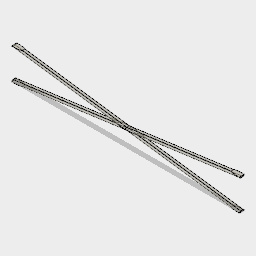
Cross braces (Autodesk Fusion 360 design; units mm, degrees)
Autodesk Fusion 360 part; units mm, degrees
sketch "Sketch1" plane through (0, 0, 0) normal (0, 0, 1) x (1, 0, 0)
  line L0 (457.0672, 59.1881) -> (558.2158, 72.9956)
  line L1 (456.2083, 65.4798) -> (534.7411, 76.2)
  line L2 (457.0672, 59.1881) -> (23.4747, 0)
  line L3 (456.2083, 65.4798) -> (0, 3.2044)
  line L4 (229.1567, 48.1231) -> (23.4747, 76.2)
  line L5 (228.2978, 41.8315) -> (0, 72.9956)
  line L6 (229.1567, 48.1231) -> (558.2158, 3.2044)
  line L7 (228.2978, 41.8315) -> (534.7411, 0)
  line L8 (23.4747, 76.2) -> (0, 76.2)
  line L9 (0, 76.2) -> (0, 72.9956)
  line L10 (0, 3.2044) -> (0, 0)
  line L11 (0, 0) -> (23.4747, 0)
  line L12 (534.7411, 76.2) -> (558.2158, 76.2)
  line L13 (558.2158, 76.2) -> (558.2158, 72.9956)
  line L14 (558.2158, 3.2044) -> (558.2158, 0)
  line L15 (558.2158, 0) -> (534.7411, 0)
  dimension "d1" = 558.2158
  dimension "d2" = 76.2
  measures "d1" distance of L10.end L14.end
  measures "d2" distance of L10.end L8.end
extrude "Extrude1" add sketch "Sketch1" along normal blind 12.7
fillet "Fillet1" radius 3.175 8 edges at (406.9245, 58.7522, 12.7) (430.3992, 20.6522, 12.7) (151.2913, 58.7522, 12.7) (430.3992, 55.5478, 12.7) (406.9245, 17.4478, 12.7) (151.2913, 17.4478, 12.7) (127.8166, 20.6522, 12.7) (127.8166, 55.5478, 12.7)
fillet "Fillet2" radius 3.175 8 edges at (127.8166, 20.6522, 0) (151.2913, 17.4478, 0) (151.2913, 58.7522, 0) (127.8166, 55.5478, 0) (406.9245, 58.7522, 0) (430.3992, 55.5478, 0) (430.3992, 20.6522, 0) (406.9245, 17.4478, 0)
